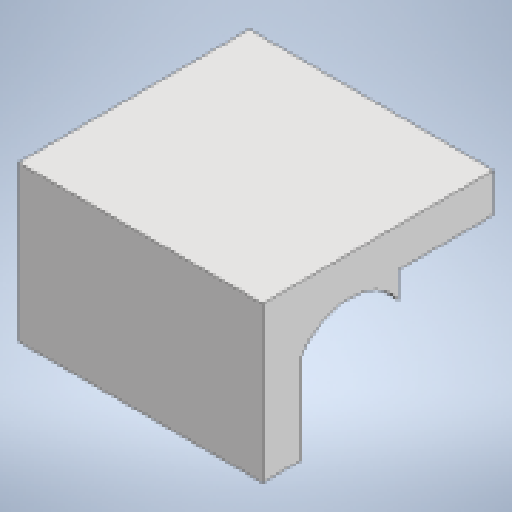
# Autodesk Inventor part: montaz_silniki
Saved by Autodesk Inventor 2023.5 (Build 275446000, 446)
## iProperties
Created: 2025-03-17
Part Number: montaz_silniki
Material: Ogólny
Document SubType Name: Modeling
Designer: kamil
Density: 1 g/cm^3
Appearance: Domyślna
Author: kamil
Autodesk Inventor part; units mm, degrees
sketch "Szkic1" plane through (0, 0, 0) normal (1, 0, 0) x (0, 1, 0)
  line L0 (0, 0) -> (12, 0)
  line L1 (12, 0) -> (12, -10)
  line L2 (16, -10) -> (16, 4)
  line L3 (16, 4) -> (0, 4)
  line L4 (0, 4) -> (0, 0)
  line L5 (12, -10) -> (16, -10)
  dimension "d0" = 12
  dimension "d1" = 10
  dimension "d2" = 4
  constraints: 12 end point, 3 perpendicular, 1 horizontal, 1 vertical, 1 other
  measures "d0" distance of L0.start L0.end
  measures "d1" distance of L0.end L1.end
  measures "d2" distance between parallel lines of L1 L2
extrude "Wyciągnięcie proste1" add sketch "Szkic1" along normal blind 9
sketch "Szkic2" plane through (0, 0, 0) normal (-1, 0, 0) x (0, 0, 1)
  arc A0 (-10.2, 9.6) -> (-19.8, 9.6) centre (-15, 6) ccw projected
  line L0 (-10, 12) -> (-10, 16) projected
  line L1 (-10, 12) -> (-10.2, 12)
  line L2 (-10.2, 12) -> (-10.2, 9.6)
  line L3 (-10, 11) -> (-10, 1) projected
  line L4 (-10, 11) -> (-10, 12)
  line L5 (-10.2, 9.6) -> (-10, 9.3166)
  line L6 (-19.8, 9.6) -> (-19.8, 16)
  line L7 (-10, 16) -> (4, 16) projected
  line L8 (-19.8, 16) -> (-10, 16)
  point P0 (0, 0)
  constraints: 12 end point, 2 perpendicular, 1 collinear, 1 horizontal, 1 point on line, 1 vertical
extrude "Wyciągnięcie proste2" add sketch "Szkic2" against normal up to surface (9 mm away)
sketch "Szkic3" plane through (9, 0, 0) normal (1, 0, 0) x (0, 0, -1)
  line L0 (0, 12) -> (10, 12) projected
  line L1 (10, 9.3166) -> (10, 12) projected
  line L2 (10.2, 9.6) -> (10, 9.3166) projected
  arc A0 (19.8, 9.6) -> (10.2, 9.6) centre (15, 6) ccw projected
  line L3 (19.8, 16) -> (19.8, 9.6) projected
  line L4 (-4, 16) -> (19.8, 16) projected
  line L5 (-4, 16) -> (-4, 0) projected
  line L6 (-4, 0) -> (0, 0) projected
  line L7 (0, 0) -> (0, 12) projected
  arc A1 (9.8, 9.6) -> (0.2, 9.6) centre (5, 6) ccw projected
  line L8 (9.8, 9.6) -> (10, 9.3166)
  line L9 (0.2, 9.6) -> (0, 9.3166)
  constraints: 4 end point, 1 point on line
ref_plane "Płaszczyzna konstrukcyjna1" through (16.1843, 0, -20) normal (-1, 0, 0) x (0, 0, 1)
extrude "Wyciągnięcie proste3" add sketch "Szkic3" along normal up to surface (7.1843 mm away)
sketch "Szkic4" plane through (16.1843, 0, 4) normal (1, 0, 0) x (0, 0, -1)
  line L0 (23, 12) -> (15, 12) projected
  arc A0 (13.8, 9.6) -> (4.2, 9.6) centre (9, 6) ccw projected
  line L1 (13.8, 9.6) -> (14, 9.3166) projected
  line L2 (14, 9.3166) -> (14.2, 9.6) projected
  arc A1 (23.8, 9.6) -> (14.2, 9.6) centre (19, 6) ccw projected
  line L3 (23.8, 9.6) -> (23.8, 16) projected
  line L4 (23.8, 16) -> (0, 16) projected
  line L5 (0, 16) -> (0, 0) projected
  line L6 (0, 0) -> (4, 0) projected
  line L7 (4, 0) -> (4, 9.3166) projected
  line L8 (4, 9.3166) -> (4.2, 9.6) projected
  line L9 (23, 12) -> (23.8, 12)
  line L10 (23.8, 9.6) -> (23.8, 16) projected
  line L11 (14, 11) -> (14, 1) projected
  line L12 (15, 12) -> (14, 12)
  line L13 (14, 12) -> (14, 11)
  point P0 (4, 0)
  constraints: 6 end point, 1 collinear, 1 horizontal, 1 perpendicular, 1 point on line
ref_plane "Płaszczyzna konstrukcyjna2" through (25.1843, 0, -20) normal (1, 0, 0) x (0, 1, 0)
extrude "Wyciągnięcie proste4" add sketch "Szkic4" along normal up to surface (9 mm away) contours L0 L12 L13 L11 L1 A0 L8 L7 L6 L5 L4 L3 L9
sketch "Szkic5" plane through (0, 9.6, -19.8) normal (0, 0, -1) x (-1, 0, 0)
  line L0 (0, 0) -> (-16.1843, 0) projected
  line L1 (0, 6.4) -> (0, 0) projected
  line L2 (0, 6.4) -> (-25.1843, 6.4) projected
  line L3 (-25.1843, 6.4) -> (-25.1843, 2.4) projected
  line L4 (-16.1843, 2.4) -> (-25.1843, 2.4) projected
  line L5 (-16.1843, 0) -> (-16.1843, 2.4) projected
  line L6 (0, -9.6) -> (-25.1843, -9.6) projected
  line L7 (0, 6.4) -> (-25.1843, 6.4) projected
  line L8 (-25.1843, 6.4) -> (0, 6.4)
  line L9 (0, 6.4) -> (0, -9.6)
  line L10 (0, -9.6) -> (-25.1843, -9.6)
  line L11 (-25.1843, -9.6) -> (-25.1843, 6.4)
  constraints: 8 end point, 2 parallel, 1 horizontal, 1 perpendicular
ref_plane "Płaszczyzna konstrukcyjna3" through (-5.8487, 1.5, -21) normal (0, 0, 1) x (1, 0, 0)
extrude "Wyciągnięcie proste5" add sketch "Szkic5" along normal up to surface (1.2 mm away)
sketch "Szkic6" plane through (0, 0, -19.8) normal (0, -1, 0) x (1, 0, 0)
  line L0 (32.6513, -1.7) -> (32.6513, -14.7) projected
  line L1 (32.1513, -15.2) -> (-5.8487, -15.2) projected
  line L2 (-5.8487, -1.2) -> (32.1513, -1.2) projected
  line L3 (-6.3487, -14.7) -> (-6.3487, -1.7) projected
  line L4 (32.6513, -1.2) -> (-6.3487, -1.2)
  line L5 (-6.3487, -1.2) -> (-6.3487, -15.2)
  line L6 (-6.3487, -15.2) -> (32.6513, -15.2)
  line L7 (32.6513, -15.2) -> (32.6513, -1.2)
  line L8 (-6.5487, -1) -> (32.8513, -1)
  line L9 (32.8513, -1) -> (32.8513, -15.4)
  line L10 (32.8513, -15.4) -> (-6.5487, -15.4)
  line L11 (-6.5487, -15.4) -> (-6.5487, -1)
  line L12 (34.8513, 1) -> (-8.5487, 1)
  line L13 (-8.5487, 1) -> (-8.5487, -17.4)
  line L14 (-8.5487, -17.4) -> (34.8513, -17.4)
  line L15 (34.8513, -17.4) -> (34.8513, 1)
  line L16 (16.1843, 0) -> (25.1843, 0) projected
  line L17 (25.1843, 0) -> (25.1843, -1.2) projected
  line L18 (25.1843, 0) -> (34.8513, 0)
  line L19 (32.8513, -1) -> (32.8513, 1)
  line L20 (25.1843, 0) -> (0, 0) projected
  line L21 (0, 0) -> (-8.5487, 0)
  line L22 (-6.5487, -1) -> (-6.5487, 1)
  point P0 (0, 19.8)
  dimension "d13" = 0.2
  dimension "d14" = 2
  constraints: 32 end point, 6 parallel, 5 perpendicular, 5 point on line, 2 horizontal, 6 other
  measures "d13" distance between parallel lines of L4 L8
  measures "d14" distance between parallel lines of L8 L12
extrude "Wyciągnięcie proste6" add sketch "Szkic6" against normal blind 1 contours L8 L9 L10 L11 | L8 L22 L21 L20 L16 L17 | L17 L18 L19 L8 | L0 L7 L6 L1 L5 L3 L4 L2 | L11 L10 L9 L19 L18 L15 L14 L13 L21 L22
sketch "Szkic7" plane through (0, 1, -19.8) normal (0, 1, 0) x (1, 0, 0)
  line L0 (0, 1.2) -> (0, 0) projected
  line L1 (25.1843, 1.2) -> (0, 1.2) projected
  line L2 (25.1843, 0) -> (25.1843, 1.2) projected
  line L3 (25.1843, 0) -> (34.8513, 0) projected
  line L4 (34.8513, 0) -> (34.8513, 17.4) projected
  line L5 (34.8513, 17.4) -> (-8.5487, 17.4) projected
  line L6 (-8.5487, 17.4) -> (-8.5487, 0) projected
  line L7 (-8.5487, 0) -> (0, 0) projected
  line L8 (32.8513, 15.4) -> (32.8513, 2)
  line L9 (-2, 2) -> (-6.5487, 2)
  line L10 (-6.5487, 2) -> (-6.5487, 15.4)
  line L11 (-6.5487, 15.4) -> (32.8513, 15.4)
  line L12 (0, 1.2) -> (-6.5487, 2)
  line L13 (32.8513, 2) -> (34.8513, 2)
  line L14 (34.8513, 0) -> (34.8513, 17.4) projected
  point P0 (0, -19.8)
  point P1 (34.8513, 2)
  dimension "d17" = 2
  constraints: 12 end point, 1 perpendicular, 1 point on line, 2 other
  measures "d17" distance between parallel lines of L4 L8
extrude "Wyciągnięcie proste7" add sketch "Szkic7" along normal blind 8 contours L0 L7 L6 L5 L4 L13 L8 L11 L10 L12
fillet "Zaokrąglenie1" radius 2 3 edges at (34.8513, 4.5, -37.2) (-8.5487, 4.5, -37.2) (-8.5487, 4.5, -19.8)
sketch "Szkic8" plane through (25.1843, 0, 4) normal (1, 0, 0) x (0, 0, -1)
  line L0 (23.8, 1) -> (25, 1) projected
  line L1 (25, 16) -> (25, 1) projected
  line L2 (0, 16) -> (25, 16) projected
  line L3 (0, 0) -> (0, 16) projected
  line L4 (4, 0) -> (0, 0) projected
  line L5 (4, 9.3166) -> (4, 0) projected
  line L6 (4.2, 9.6) -> (4, 9.3166) projected
  arc A0 (13.8, 9.6) -> (4.2, 9.6) centre (9, 6) ccw projected
  line L7 (14, 9.3166) -> (13.8, 9.6) projected
  line L8 (14, 12) -> (14, 9.3166) projected
  line L9 (23.8, 12) -> (14, 12) projected
  line L10 (23.8, 12) -> (23.8, 1) projected
  line L11 (23.8, 12) -> (14, 12) projected
  line L12 (14, 12) -> (14, 16)
  line L13 (0, 16) -> (25, 16) projected
  point P0 (4, 0)
  point P1 (14, 16)
  constraints: 2 end point, 1 perpendicular, 1 point on line
ref_plane "Płaszczyzna konstrukcyjna4" through (27.1843, 3.25, -7.75) normal (1, 0, 0) x (0, 1, 0)
extrude "Wyciągnięcie proste8" add sketch "Szkic8" along normal up to surface (2 mm away) contours L8 L7 A0 L6 L5 L4 L3 L2 L12
sketch "Szkic9" plane through (27.1843, 0, 4) normal (1, 0, 0) x (0, 0, -1)
  circle A0 centre (9, 6) radius 2.75 projected
  arc A1 (13.8, 9.6) -> (4.2, 9.6) centre (9, 6) ccw projected
  line L0 (14, 9.3166) -> (14, 0)
  line L1 (4, 9.3166) -> (4, 0) projected
  line L2 (4.2, 9.6) -> (4, 9.3166) projected
  line L3 (4, 0) -> (14, 0)
  line L4 (14, 9.3166) -> (13.8, 9.6) projected
  constraints: 4 end point, 1 horizontal, 1 vertical
extrude "Wyciągnięcie proste9" add sketch "Szkic9" against normal blind 0.8
sketch "Szkic10" plane through (27.1843, 0, 4) normal (1, 0, 0) x (0, 0, -1)
  circle A0 centre (9, 6) radius 1.47 projected
  circle A1 centre (9, 6) radius 2.75 projected
  line L0 (0, 0) -> (0, 16) projected
  line L1 (0, 0) -> (14, 0) projected
  line L2 (14, 16) -> (14, 0) projected
  line L3 (0, 16) -> (14, 16) projected
  point P0 (4, 0)
extrude "Wyciągnięcie proste10" add sketch "Szkic10" along normal blind 3.2 contours A1 | L0 L3 L2 L1
sketch "Szkic11" plane through (26.3843, 0, 4) normal (-1, 0, 0) x (0, 0, 1)
  circle A0 centre (-9, 6) radius 2.75 projected
  circle A1 centre (-9, 6) radius 2.95
  point P0 (-4, 0)
  dimension "d27" = 0.2
  constraints: 1 centre point
  measures "d27" radial gap between concentric circles of A0 A1
extrude "Wyciągnięcie proste11" cut sketch "Szkic11" against normal up to surface (0.8 mm away) contours A0 | A1
sketch "Szkic12" plane through (27.1843, 6, -5) normal (-1, 0, 0) x (0, 0, 1)
  circle A0 centre (0, 0) radius 1.47 projected
  circle A1 centre (0, 0) radius 1.67
  point P0 (5, -6)
  dimension "d30" = 0.2
  constraints: 1 centre point
  measures "d30" radial gap between concentric circles of A0 A1
extrude "Wyciągnięcie proste12" cut sketch "Szkic12" against normal through all contours A0 | A1
